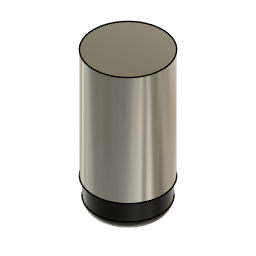
KS5N (Autodesk Fusion 360 design; units mm, degrees)
Autodesk Fusion 360 part; units mm, degrees
note: some values were not read from the file. Chosen so that the rebuilt part matches the saved one: which bodies a step acts on.
sketch "スケッチ1" plane through (0, 0, 0) normal (0, 0, 1) x (1, 0, 0)
  circle A0 centre (0, 0) radius 18
  dimension "d1" = 36
  constraint coincident A0.centre origin
  measures "d1" diameter of A0
extrude "押し出し1" add sketch "スケッチ1" along normal blind 57.1 makes body 1
sketch "スケッチ2" plane through (0, 0, 0) normal (0, 0, -1) x (1, 0, 0)
  circle A0 centre (0, 0) radius 18
  circle A1 centre (0, 0) radius 17
  dimension "d4" = 34
  constraint coincident A0.centre A1.centre
  measures "d4" diameter of A1
extrude "押し出し2" add sketch "スケッチ2" along normal blind 14 contours A1 bodies 1
fillet "フィレット1" radius 5 1 edges at (-15.8496, 6.1475, -14) on bodies 1
split "分割1" by plane through (0, 0, 0) normal (0, 0, -1) bodies 1 makes body 2 at (16.9789, 0.8474, -6)
copy_body "ボディ -> コンポーネント1" bodies 1 removing the originals makes body 3 in component "Component"
copy_body "ボディ -> コンポーネント2" bodies 2 removing the originals makes body 4 in component "Component'"
component "Component'" placed x (1, 0, 0) y (0, 1, 0) z (0, 0, 1) at (0, 0, 0)
component "Component" placed x (1, 0, 0) y (0, 1, 0) z (0, 0, 1) at (0, 0, 0)
